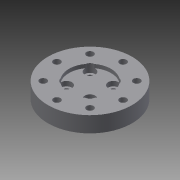
# Autodesk Inventor part: Plate
Saved by Autodesk Inventor 2013 (Build 170138000, 138)
## iProperties
Created: 2013-01-29
Part Number: Plate
Material: Generic
Document SubType Name: Modeling
Designer: Mahisorn
Density: 1 g/cm^3
Author: Mahisorn
Autodesk Inventor part; units mm, degrees
ref_plane "YZ Plane" through (0, 0, 0) normal (1, 0, 0) x (0, 1, 0)
ref_plane "XZ Plane" through (0, 0, 0) normal (0, 1, 0) x (-1, 0, 0)
ref_plane "XY Plane" through (0, 0, 0) normal (0, 0, 1) x (1, 0, 0)
sketch "Sketch1" plane through (0, 0, 0) normal (0, 1, 0) x (-1, 0, 0)
  circle A0 centre (0, 0) radius 40
  circle A1 centre (0, 0) radius 21
  point P0 (11.1369, 11.1369)
  point P1 (-11.1369, 11.1369)
  point P2 (-11.1369, -11.1369)
  point P3 (11.1369, -11.1369)
  dimension "d0" = 80
  dimension "d2" = 15.75
  dimension "d5" = 360
  dimension "d16" = 42
  constraints: 2 centre point, 2 coincident, 5 other
  measures "d0" diameter of A0
  measures "d2" distance of point (0, 0) point (11.137, 11.137)
  measures "d16" diameter of A1
extrude "Extrusion1" add sketch "Sketch1" against normal blind 15 contours A0 | A1
hole "Hole1" at (-11.1369, 0, 11.1369) at (11.1369, 0, 11.1369) at (11.1369, 0, -11.1369) at (-11.1369, 0, -11.1369) direction (0, -1, 0) diameter 5.5 end through all counterbore diameter 10 counterbore depth 8.5 clearance for "Socket Head Cap Screw" size "M5" standard "Ansi Metric M Profile"
extrude "Extrusion2" cut sketch "Sketch1" against normal blind 3.5 contours A1
sketch "Sketch2" plane through (0, -15, 0) normal (0, -1, 0) x (1, 0, 0)
  circle A0 centre (0, 0) radius 40 projected
  circle A1 centre (0, 0) radius 20
  point P0 (31.5, 0)
  point P1 (22.2739, 22.2739)
  point P2 (0, 31.5)
  point P3 (-22.2739, 22.2739)
  point P4 (-31.5, 0)
  point P5 (-22.2739, -22.2739)
  point P6 (0, -31.5)
  point P7 (22.2739, -22.2739)
  point P8 (23.097, 9.5671)
  dimension "d25" = 31.5
  dimension "d26" = 40
  dimension "d29" = 360
  dimension "d38" = 25
  constraints: 1 centre point, 1 coincident, 1 other
  measures "d25" distance of A0.centre point (31.5, 0)
  measures "d26" diameter of A1
  measures "d38" distance of A0.centre point (23.097, 9.567)
hole "Hole2" at (22.2739, -15, 22.2739) at (31.5, -15, 0) at (22.2739, -15, -22.2739) at (0, -15, -31.5) at (-22.2739, -15, -22.2739) at (-31.5, -15, 0) at (-22.2739, -15, 22.2739) at (0, -15, 31.5) direction (0, 1, 0) diameter 6.6 end through all clearance for "Hex Head Bolt" size "M6" standard "Ansi Metric M Profile"
body "Solid1"
